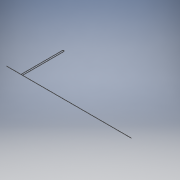
# Autodesk Inventor part: BeltMain
Saved by Autodesk Inventor 2017 (Build 210142000, 142)
## iProperties
Created: 2016-12-13
Part Number: BeltMain
Material: Rubber
Document SubType Name: Modeling
Designer: umr
Density: 0.93 g/cm^3
Appearance: Rubber - Black
Mass: 1.70553 g
Surface Area: 44.7756 cm^2
Volume: 1.8339 cm^3
Author: umr
Autodesk Inventor part; units mm, degrees
ref_plane "YZ Plane" through (0, 0, 0) normal (1, 0, 0) x (0, 1, 0)
ref_plane "XZ Plane" through (0, 0, 0) normal (0, 1, 0) x (-1, 0, 0)
ref_plane "XY Plane" through (0, 0, 0) normal (0, 0, 1) x (1, 0, 0)
sketch "Sketch2" plane through (0, 0, 0) normal (0, 0, 1) x (1, 0, 0)
  line L0 (0, 0) -> (2420, 0)
  line L1 (2420, 0) -> (2420, 3)
  line L2 (2420, 3) -> (0, 3)
  line L3 (0, 3) -> (0, 0)
  line L4 (307, 3) -> (307, 803)
  line L5 (307, 803) -> (310, 803)
  line L6 (310, 803) -> (310, 3)
  line L7 (310, 803) -> (1110, 803) construction
  line L8 (277, 3) -> (277, 803)
  line L9 (277, 803) -> (280, 803)
  line L10 (280, 803) -> (280, 3)
  line L11 (310, 806) -> (310, 803)
  line L12 (310, 3) -> (307, 3)
  line L13 (277, 3) -> (280, 3)
  line L14 (277, 3) -> (280, 3)
  arc A0 (310, 803) -> (277, 803) centre (293.5, 803) ccw
  arc A1 (307, 803) -> (280, 803) centre (293.5, 803) ccw
  line L15 (277, 803) -> (280, 803)
  line L16 (307, 803) -> (310, 803)
  dimension "d16" = 2420
  dimension "d17" = 3
  dimension "d18" = 90
  dimension "d21" = 800
  dimension "d22" = 3
  dimension "d23" = 90
  dimension "d24" = 90
  dimension "d25" = 2110
  dimension "d28" = 30
  constraints: 34 end point, 5 perpendicular, 4 horizontal, 4 point on circle, 4 point on line, 3 collinear, 2 centre point, 1 coincident, 1 parallel, 1 tangent, 7 other
  measures "d16" distance of L0.start L0.end
  measures "d17" distance of L0.end L1.end
  measures "d18" angle of L2 L1
  measures "d21" distance of L4.start L4.end
  measures "d22" distance of L5.end L4.end
  measures "d23" angle of L4 L5
  measures "d24" angle of L6 L7
  measures "d25" distance from line of L6 L1.end
  measures "d28" distance of L4.start L8.start
extrude "Extrusion2" add sketch "Sketch2" along normal blind 6 contours L3 L2 L1 L0 | L8 L9 L10 L2 | L2 L4 L5 L6 | A0 L5 A1 L9
body "Solid2"
